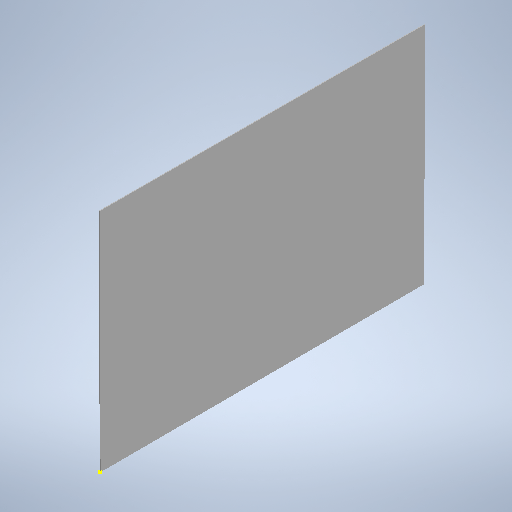
# Autodesk Inventor part: floar
Saved by Autodesk Inventor 2025.2 (Build 292293000, 293)
## iProperties
Created: 2025-06-25
Part Number: floar
Material: 一般
Document SubType Name: Modeling
Designer: naka6
Density: 1 g/cm^3
Appearance: 既定
Author: naka6
Autodesk Inventor part; units mm, degrees
ref_plane "YZ Plane" through (0, 0, 0) normal (1, 0, 0) x (0, 1, 0)
ref_plane "XZ Plane" through (0, 0, 0) normal (0, 1, 0) x (-1, 0, 0)
ref_plane "XY Plane" through (0, 0, 0) normal (0, 0, 1) x (1, 0, 0)
sketch "スケッチ1" plane through (0, 0, 0) normal (1, 0, 0) x (0, 1, 0)
  line L0 (0, 0) -> (2847.2316, 0)
  line L1 (2847.2316, 0) -> (2847.2316, -4099.8518)
  line L2 (2847.2316, -4099.8518) -> (0, -4099.8518)
  line L3 (0, -4099.8518) -> (0, 0)
  constraints: 8 end point, 2 parallel, 1 horizontal, 1 perpendicular
extrude "押し出し1" add sketch "スケッチ1" along normal blind 10
sketch "スケッチ3" plane through (0, 0, 0) normal (-1, 0, 0) x (0, 0, 1)
  line L0 (-2182.6632, 1388.0504) -> (-2013.9556, 1388.0504) construction
  line L1 (-2013.9556, 1388.0504) -> (-2013.9556, 1293.1524) construction
  line L2 (-2013.9556, 1293.1524) -> (-2182.6632, 1293.1524) construction
  line L3 (-2182.6632, 1293.1524) -> (-2182.6632, 1388.0504) construction
  line L4 (-2182.6632, 1482.9484) -> (-2013.9556, 1482.9484) construction
  line L5 (-2013.9556, 1482.9484) -> (-2013.9556, 1388.0504) construction
  line L6 (-2013.9556, 1388.0504) -> (-2182.6632, 1388.0504) construction
  line L7 (-2182.6632, 1388.0504) -> (-2182.6632, 1482.9484) construction
  line L8 (-2351.3664, 1388.0424) -> (-2182.6588, 1388.0424) construction
  line L9 (-2182.6588, 1388.0424) -> (-2182.6588, 1293.1444) construction
  line L10 (-2182.6588, 1293.1444) -> (-2351.3664, 1293.1444) construction
  line L11 (-2351.3664, 1293.1444) -> (-2351.3664, 1388.0424) construction
  line L12 (-2182.6588, 1482.9403) -> (-2182.6588, 1388.0424) construction
  line L13 (-2351.3664, 1388.0424) -> (-2351.3664, 1482.9403) construction
  line L14 (-2182.6588, 1388.0424) -> (-2351.3664, 1388.0424) construction
  line L15 (-2351.3664, 1482.9403) -> (-2182.6588, 1482.9403) construction
  line L16 (-2182.6672, 1293.18) -> (-2013.9597, 1293.18) construction
  line L17 (-2013.9597, 1293.18) -> (-2013.9597, 1198.282) construction
  line L18 (-2013.9597, 1198.282) -> (-2182.6672, 1198.282) construction
  line L19 (-2182.6672, 1198.282) -> (-2182.6672, 1293.18) construction
  line L20 (-2351.3748, 1293.18) -> (-2182.6672, 1293.18) construction
  line L21 (-2182.6672, 1293.18) -> (-2182.6672, 1198.282) construction
  line L22 (-2182.6672, 1198.282) -> (-2351.3748, 1198.282) construction
  line L23 (-2351.3748, 1198.282) -> (-2351.3748, 1293.18) construction
  line L24 (-2182.6633, 1577.8359) -> (-2013.9602, 1577.8439) construction
  line L25 (-2013.9602, 1577.8439) -> (-2013.9556, 1482.9484) construction
  line L26 (-2013.9556, 1482.9484) -> (-2182.6588, 1482.9403) construction
  line L27 (-2182.6588, 1482.9403) -> (-2182.6633, 1577.8359) construction
  line L28 (-2351.3664, 1577.8383) -> (-2182.6588, 1577.8383) construction
  line L29 (-2182.6588, 1577.8383) -> (-2182.6588, 1482.9403) construction
  line L30 (-2182.6588, 1482.9403) -> (-2351.3664, 1482.9403) construction
  line L31 (-2351.3664, 1482.9403) -> (-2351.3664, 1577.8383) construction
  point P0 (0, 0)
  constraints: 9 coincident, 16 other
